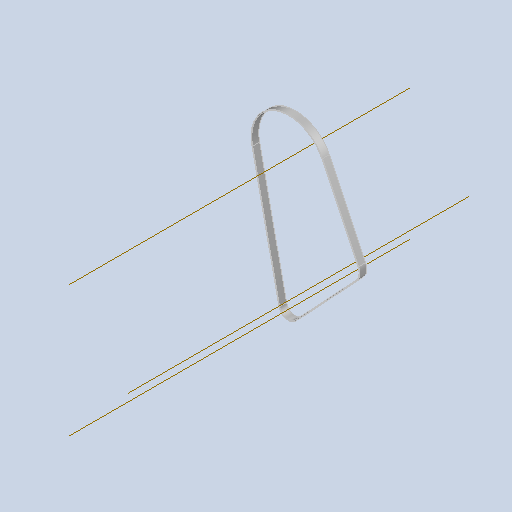
# Autodesk Inventor part: Synchronous Belt
Saved by Autodesk Inventor 2024 (Build 280153000, 153)
## iProperties
Created: 2024-01-05
Part Number: Synchronous Belt
Material: Rubber
Document SubType Name: Modeling
Designer: MaartenGeorgesBuelen
Density: 1 g/cm^3
Appearance: Rubber - Black - Version 1.1
CustomPartVersion: 1
Author: MaartenGeorgesBuelen
Autodesk Inventor part; units mm, degrees
sketch "Sketch Path" plane through (0, 0, 0) normal (0, 0, 1) x (1, 0, 0)
  arc A0 (-7.7801, -1.672) -> (5.8114, -5.4363) centre (0, 0) ccw
  arc A1 (28.9379, 126.2523) -> (-30.8718, 105.775) centre (0.2486, 112.4632) ccw
  arc A2 (58.2507, 50.621) -> (59.9518, 61.7255) centre (50.9864, 57.4164) ccw
  line L0 (58.2507, 50.621) -> (5.8114, -5.4363)
  line L1 (-7.7801, -1.672) -> (-30.8718, 105.775)
  line L2 (28.9379, 126.2523) -> (59.9518, 61.7255)
  constraints: 6 end point, 6 point on circle, 3 centre point
ref_plane "Cross Section Plane" through (5.8114, -5.4363, 0) normal (0.6831, 0.7303, 0) x (0, 0, 1)
ref_plane "Work Plane2" through (0, 0, 0) normal (-1, 0, 0) x (0, 0, 1)
ref_plane "Work Plane3" through (0.2486, 112.4632, 0) normal (0.155, -0.9879, 0) x (0, 0, 1)
ref_plane "Work Plane4" through (50.9864, 57.4164, 0) normal (-0.4137, 0.9104, 0) x (0, 0, 1)
sketch "Cross Section" plane through (5.8114, -5.4363, 0) normal (0.6831, 0.7303, 0) x (0, 0, 1)
  line L0 (-3, 0.3) -> (3, 0.3)
  line L1 (3, 0.3) -> (3, -0.3)
  line L2 (3, -0.3) -> (-3, -0.3)
  line L3 (-3, -0.3) -> (-3, 0.3)
  line L4 (-3, 0) -> (3, 0) construction
  point P0 (0, 0)
  point P1 (0, 0)
  dimension "d0" = 6
  dimension "d4" = 0.3
  dimension "d5" = 0.3
  constraints: 10 end point, 3 midpoint, 2 parallel, 1 coincident, 1 horizontal, 1 perpendicular, 1 other
  measures "d0" distance between parallel lines of L1 L3
  measures "d4" distance between parallel lines of L2 L4
  measures "d5" distance between parallel lines of L4 L0
sweep "Belt" add profiles "Cross Section" path "Sketch Path"
equation "\"d0\" = da_B"
equation "\"d4\" = da_a"
equation "\"d5\" = da_a2"
equation "\"da_B\" = 6"
equation "\"da_pb\" = 2.5"
equation "\"da_a\" = 0.3"
equation "\"da_S\" = 1.5"
equation "\"da_Beta\" = 20deg"
equation "\"da_Ht\" = 0.7"
equation "\"da_H\" = 1.3"
equation "\"da_a2\" = 0.3"
body "Solid1"
